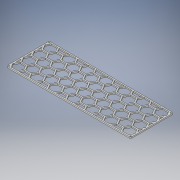
# Autodesk Inventor part: plate
Saved by Autodesk Inventor 2019 (Build 230136000, 136)
## iProperties
Created: 2019-01-24
Part Number: plate
Material: Generic
Document SubType Name: Modeling
Designer: Andrew
Density: 1 g/cm^3
Appearance: Default
Author: Andrew
Autodesk Inventor part; units mm, degrees
ref_plane "YZ Plane" through (0, 0, 0) normal (1, 0, 0) x (0, 1, 0)
ref_plane "XZ Plane" through (0, 0, 0) normal (0, 1, 0) x (-1, 0, 0)
ref_plane "XY Plane" through (0, 0, 0) normal (0, 0, 1) x (1, 0, 0)
sketch "Sketch1" plane through (0, 0, 0) normal (0, 1, 0) x (-1, 0, 0)
  line L0 (290.7004, 97.1993) -> (290.7004, 3)
  arc A0 (287.7004, 0) -> (290.7004, 3) centre (287.7004, 3) ccw
  arc A1 (290.7004, 97.1993) -> (287.7004, 100.1993) centre (287.7004, 97.1993) ccw
  line L1 (3, 0) -> (287.7004, 0)
  line L2 (0, 97.1993) -> (0, 3)
  line L3 (287.7004, 100.1993) -> (3, 100.1993)
  arc A2 (3, 100.1993) -> (0, 97.1993) centre (3, 97.1993) ccw
  circle A3 centre (287.7004, 97.1993) radius 1.5
  circle A4 centre (3, 97.1993) radius 1.5
  circle A5 centre (3, 3) radius 1.5
  circle A6 centre (287.7004, 3) radius 1.5
  line L4 (3, 88.615) -> (3, 86.7338)
  line L5 (7.9562, 3) -> (22.4187, 3)
  line L6 (287.7004, 88.615) -> (287.7004, 86.7338)
  line L7 (282.7442, 97.1993) -> (268.2817, 97.1993)
  arc A7 (0, 3) -> (3, 0) centre (3, 3) ccw
  line L8 (30.516, 86.1744) -> (24.1507, 75.1495)
  line L9 (30.516, 86.1744) -> (43.2465, 86.1744)
  line L10 (43.2465, 86.1744) -> (49.6117, 75.1495)
  line L11 (49.6117, 75.1495) -> (43.2465, 64.1246)
  line L12 (30.516, 64.1246) -> (43.2465, 64.1246)
  line L13 (24.1507, 75.1495) -> (30.516, 64.1246)
  line L14 (52.2098, 73.6495) -> (45.8445, 62.6246)
  line L15 (45.8445, 62.6246) -> (52.2098, 51.5997)
  line L16 (71.3055, 62.6246) -> (64.9402, 51.5997)
  line L17 (64.9402, 73.6495) -> (71.3055, 62.6246)
  line L18 (52.2098, 51.5997) -> (64.9402, 51.5997)
  line L19 (52.2098, 73.6495) -> (64.9402, 73.6495)
  line L20 (73.9036, 86.1744) -> (67.5383, 75.1495)
  line L21 (67.5383, 75.1495) -> (73.9036, 64.1246)
  line L22 (92.9993, 75.1495) -> (86.634, 64.1246)
  line L23 (86.634, 86.1744) -> (92.9993, 75.1495)
  line L24 (73.9036, 64.1246) -> (86.634, 64.1246)
  line L25 (73.9036, 86.1744) -> (86.634, 86.1744)
  line L26 (95.5974, 73.6495) -> (89.2321, 62.6246)
  line L27 (89.2321, 62.6246) -> (95.5974, 51.5997)
  line L28 (114.6931, 62.6246) -> (108.3278, 51.5997)
  line L29 (108.3278, 73.6495) -> (114.6931, 62.6246)
  line L30 (95.5974, 51.5997) -> (108.3278, 51.5997)
  line L31 (95.5974, 73.6495) -> (108.3278, 73.6495)
  line L32 (73.9036, 61.1246) -> (67.5383, 50.0997)
  line L33 (67.5383, 50.0997) -> (73.9036, 39.0747)
  line L34 (92.9993, 50.0997) -> (86.634, 39.0747)
  line L35 (86.634, 61.1246) -> (92.9993, 50.0997)
  line L36 (73.9036, 39.0747) -> (86.634, 39.0747)
  line L37 (73.9036, 61.1246) -> (86.634, 61.1246)
  line L38 (52.2098, 48.5997) -> (45.8445, 37.5747)
  line L39 (45.8445, 37.5747) -> (52.2098, 26.5498)
  line L40 (71.3055, 37.5747) -> (64.9402, 26.5498)
  line L41 (64.9402, 48.5997) -> (71.3055, 37.5747)
  line L42 (52.2098, 26.5498) -> (64.9402, 26.5498)
  line L43 (52.2098, 48.5997) -> (64.9402, 48.5997)
  line L44 (73.9036, 36.0747) -> (67.5383, 25.0498)
  line L45 (67.5383, 25.0498) -> (73.9036, 14.0249)
  line L46 (92.9993, 25.0498) -> (86.634, 14.0249)
  line L47 (86.634, 36.0747) -> (92.9993, 25.0498)
  line L48 (73.9036, 14.0249) -> (86.634, 14.0249)
  line L49 (73.9036, 36.0747) -> (86.634, 36.0747)
  line L50 (95.5974, 48.5997) -> (89.2321, 37.5747)
  line L51 (89.2321, 37.5747) -> (95.5974, 26.5498)
  line L52 (114.6931, 37.5747) -> (108.3278, 26.5498)
  line L53 (108.3278, 48.5997) -> (114.6931, 37.5747)
  line L54 (95.5974, 26.5498) -> (108.3278, 26.5498)
  line L55 (95.5974, 48.5997) -> (108.3278, 48.5997)
  line L56 (117.2911, 61.1246) -> (110.9259, 50.0997)
  line L57 (110.9259, 50.0997) -> (117.2911, 39.0747)
  line L58 (136.3869, 50.0997) -> (130.0216, 39.0747)
  line L59 (130.0216, 61.1246) -> (136.3869, 50.0997)
  line L60 (117.2911, 39.0747) -> (130.0216, 39.0747)
  line L61 (117.2911, 61.1246) -> (130.0216, 61.1246)
  line L62 (138.9849, 73.6495) -> (132.6197, 62.6246)
  line L63 (132.6197, 62.6246) -> (138.9849, 51.5997)
  line L64 (158.0807, 62.6246) -> (151.7154, 51.5997)
  line L65 (151.7154, 73.6495) -> (158.0807, 62.6246)
  line L66 (138.9849, 51.5997) -> (151.7154, 51.5997)
  line L67 (138.9849, 73.6495) -> (151.7154, 73.6495)
  line L68 (160.6787, 61.1246) -> (154.3135, 50.0997)
  line L69 (154.3135, 50.0997) -> (160.6787, 39.0747)
  line L70 (179.7744, 50.0997) -> (173.4092, 39.0747)
  line L71 (173.4092, 61.1246) -> (179.7744, 50.0997)
  line L72 (160.6787, 39.0747) -> (173.4092, 39.0747)
  line L73 (160.6787, 61.1246) -> (173.4092, 61.1246)
  line L74 (138.9849, 48.5997) -> (132.6197, 37.5747)
  line L75 (132.6197, 37.5747) -> (138.9849, 26.5498)
  line L76 (158.0807, 37.5747) -> (151.7154, 26.5498)
  line L77 (151.7154, 48.5997) -> (158.0807, 37.5747)
  line L78 (138.9849, 26.5498) -> (151.7154, 26.5498)
  line L79 (138.9849, 48.5997) -> (151.7154, 48.5997)
  line L80 (117.2911, 36.0747) -> (110.9259, 25.0498)
  line L81 (110.9259, 25.0498) -> (117.2911, 14.0249)
  line L82 (136.3869, 25.0498) -> (130.0216, 14.0249)
  line L83 (130.0216, 36.0747) -> (136.3869, 25.0498)
  line L84 (117.2911, 14.0249) -> (130.0216, 14.0249)
  line L85 (117.2911, 36.0747) -> (130.0216, 36.0747)
  line L86 (160.6787, 36.0747) -> (154.3135, 25.0498)
  line L87 (154.3135, 25.0498) -> (160.6787, 14.0249)
  line L88 (179.7744, 25.0498) -> (173.4092, 14.0249)
  line L89 (173.4092, 36.0747) -> (179.7744, 25.0498)
  line L90 (160.6787, 14.0249) -> (173.4092, 14.0249)
  line L91 (160.6787, 36.0747) -> (173.4092, 36.0747)
  line L92 (182.3725, 48.5997) -> (176.0073, 37.5747)
  line L93 (176.0073, 37.5747) -> (182.3725, 26.5498)
  line L94 (201.4682, 37.5747) -> (195.103, 26.5498)
  line L95 (195.103, 48.5997) -> (201.4682, 37.5747)
  line L96 (182.3725, 26.5498) -> (195.103, 26.5498)
  line L97 (182.3725, 48.5997) -> (195.103, 48.5997)
  line L98 (182.3725, 73.6495) -> (176.0073, 62.6246)
  line L99 (176.0073, 62.6246) -> (182.3725, 51.5997)
  line L100 (201.4682, 62.6246) -> (195.103, 51.5997)
  line L101 (195.103, 73.6495) -> (201.4682, 62.6246)
  line L102 (182.3725, 51.5997) -> (195.103, 51.5997)
  line L103 (182.3725, 73.6495) -> (195.103, 73.6495)
  line L104 (160.6787, 86.1744) -> (154.3135, 75.1495)
  line L105 (154.3135, 75.1495) -> (160.6787, 64.1246)
  line L106 (179.7744, 75.1495) -> (173.4092, 64.1246)
  line L107 (173.4092, 86.1744) -> (179.7744, 75.1495)
  line L108 (160.6787, 64.1246) -> (173.4092, 64.1246)
  line L109 (160.6787, 86.1744) -> (173.4092, 86.1744)
  line L110 (204.0663, 86.1744) -> (197.7011, 75.1495)
  line L111 (197.7011, 75.1495) -> (204.0663, 64.1246)
  line L112 (223.162, 75.1495) -> (216.7968, 64.1246)
  line L113 (216.7968, 86.1744) -> (223.162, 75.1495)
  line L114 (204.0663, 64.1246) -> (216.7968, 64.1246)
  line L115 (204.0663, 86.1744) -> (216.7968, 86.1744)
  line L116 (204.0663, 61.1246) -> (197.7011, 50.0997)
  line L117 (197.7011, 50.0997) -> (204.0663, 39.0747)
  line L118 (223.162, 50.0997) -> (216.7968, 39.0747)
  line L119 (216.7968, 61.1246) -> (223.162, 50.0997)
  line L120 (204.0663, 39.0747) -> (216.7968, 39.0747)
  line L121 (204.0663, 61.1246) -> (216.7968, 61.1246)
  line L122 (225.7601, 73.6495) -> (219.3949, 62.6246)
  line L123 (219.3949, 62.6246) -> (225.7601, 51.5997)
  line L124 (244.8558, 62.6246) -> (238.4906, 51.5997)
  line L125 (238.4906, 73.6495) -> (244.8558, 62.6246)
  line L126 (225.7601, 51.5997) -> (238.4906, 51.5997)
  line L127 (225.7601, 73.6495) -> (238.4906, 73.6495)
  line L128 (225.7601, 48.5997) -> (219.3949, 37.5747)
  line L129 (219.3949, 37.5747) -> (225.7601, 26.5498)
  line L130 (244.8558, 37.5747) -> (238.4906, 26.5498)
  line L131 (238.4906, 48.5997) -> (244.8558, 37.5747)
  line L132 (225.7601, 26.5498) -> (238.4906, 26.5498)
  line L133 (225.7601, 48.5997) -> (238.4906, 48.5997)
  line L134 (204.0663, 36.0747) -> (197.7011, 25.0498)
  line L135 (197.7011, 25.0498) -> (204.0663, 14.0249)
  line L136 (223.162, 25.0498) -> (216.7968, 14.0249)
  line L137 (216.7968, 36.0747) -> (223.162, 25.0498)
  line L138 (204.0663, 14.0249) -> (216.7968, 14.0249)
  line L139 (204.0663, 36.0747) -> (216.7968, 36.0747)
  line L140 (247.4539, 36.0747) -> (241.0887, 25.0498)
  line L141 (241.0887, 25.0498) -> (247.4539, 14.0249)
  line L142 (266.5496, 25.0498) -> (260.1844, 14.0249)
  line L143 (260.1844, 36.0747) -> (266.5496, 25.0498)
  line L144 (247.4539, 14.0249) -> (260.1844, 14.0249)
  line L145 (247.4539, 36.0747) -> (260.1844, 36.0747)
  line L146 (247.4539, 61.1246) -> (241.0887, 50.0997)
  line L147 (241.0887, 50.0997) -> (247.4539, 39.0747)
  line L148 (266.5496, 50.0997) -> (260.1844, 39.0747)
  line L149 (260.1844, 61.1246) -> (266.5496, 50.0997)
  line L150 (247.4539, 39.0747) -> (260.1844, 39.0747)
  line L151 (247.4539, 61.1246) -> (260.1844, 61.1246)
  line L152 (247.4539, 86.1744) -> (241.0887, 75.1495)
  line L153 (241.0887, 75.1495) -> (247.4539, 64.1246)
  line L154 (266.5496, 75.1495) -> (260.1844, 64.1246)
  line L155 (260.1844, 86.1744) -> (266.5496, 75.1495)
  line L156 (247.4539, 64.1246) -> (260.1844, 64.1246)
  line L157 (247.4539, 86.1744) -> (260.1844, 86.1744)
  line L158 (30.516, 61.1246) -> (24.1507, 50.0997)
  line L159 (24.1507, 50.0997) -> (30.516, 39.0747)
  line L160 (49.6117, 50.0997) -> (43.2465, 39.0747)
  line L161 (43.2465, 61.1246) -> (49.6117, 50.0997)
  line L162 (30.516, 39.0747) -> (43.2465, 39.0747)
  line L163 (30.516, 61.1246) -> (43.2465, 61.1246)
  line L164 (30.516, 36.0747) -> (24.1507, 25.0498)
  line L165 (24.1507, 25.0498) -> (30.516, 14.0249)
  line L166 (49.6117, 25.0498) -> (43.2465, 14.0249)
  line L167 (43.2465, 36.0747) -> (49.6117, 25.0498)
  line L168 (30.516, 14.0249) -> (43.2465, 14.0249)
  line L169 (30.516, 36.0747) -> (43.2465, 36.0747)
  line L170 (8.8222, 73.6495) -> (3, 63.5652)
  line L171 (3, 61.684) -> (8.8222, 51.5997)
  line L172 (27.9179, 62.6246) -> (21.5527, 51.5997)
  line L173 (21.5527, 73.6495) -> (27.9179, 62.6246)
  line L174 (8.8222, 51.5997) -> (21.5527, 51.5997)
  line L175 (8.8222, 73.6495) -> (21.5527, 73.6495)
  line L176 (7.9562, 97.1993) -> (3, 88.615)
  line L177 (3, 86.7338) -> (8.8222, 76.6495)
  line L178 (27.9179, 87.6744) -> (21.5527, 76.6495)
  line L179 (22.4187, 97.1993) -> (27.9179, 87.6744)
  line L180 (8.8222, 76.6495) -> (21.5527, 76.6495)
  line L181 (8.8222, 48.5997) -> (3, 38.5153)
  line L182 (3, 36.6342) -> (8.8222, 26.5498)
  line L183 (27.9179, 37.5747) -> (21.5527, 26.5498)
  line L184 (21.5527, 48.5997) -> (27.9179, 37.5747)
  line L185 (8.8222, 26.5498) -> (21.5527, 26.5498)
  line L186 (8.8222, 48.5997) -> (21.5527, 48.5997)
  line L187 (25.8828, 97.1993) -> (30.516, 89.1744)
  line L188 (47.8796, 97.1993) -> (43.2465, 89.1744)
  line L189 (30.516, 89.1744) -> (43.2465, 89.1744)
  line L190 (69.2704, 97.1993) -> (73.9036, 89.1744)
  line L191 (91.2672, 97.1993) -> (86.634, 89.1744)
  line L192 (73.9036, 89.1744) -> (86.634, 89.1744)
  line L193 (112.658, 97.1993) -> (117.2911, 89.1744)
  line L194 (134.6548, 97.1993) -> (130.0216, 89.1744)
  line L195 (117.2911, 89.1744) -> (130.0216, 89.1744)
  line L196 (156.0455, 97.1993) -> (160.6787, 89.1744)
  line L197 (178.0424, 97.1993) -> (173.4092, 89.1744)
  line L198 (160.6787, 89.1744) -> (173.4092, 89.1744)
  line L199 (199.4331, 97.1993) -> (204.0663, 89.1744)
  line L200 (221.43, 97.1993) -> (216.7968, 89.1744)
  line L201 (204.0663, 89.1744) -> (216.7968, 89.1744)
  line L202 (242.8207, 97.1993) -> (247.4539, 89.1744)
  line L203 (264.8176, 97.1993) -> (260.1844, 89.1744)
  line L204 (247.4539, 89.1744) -> (260.1844, 89.1744)
  line L205 (224.8941, 97.1993) -> (219.3949, 87.6744)
  line L206 (219.3949, 87.6744) -> (225.7601, 76.6495)
  line L207 (244.8558, 87.6744) -> (238.4906, 76.6495)
  line L208 (239.3566, 97.1993) -> (244.8558, 87.6744)
  line L209 (225.7601, 76.6495) -> (238.4906, 76.6495)
  line L210 (181.5065, 97.1993) -> (176.0073, 87.6744)
  line L211 (176.0073, 87.6744) -> (182.3725, 76.6495)
  line L212 (201.4682, 87.6744) -> (195.103, 76.6495)
  line L213 (195.969, 97.1993) -> (201.4682, 87.6744)
  line L214 (182.3725, 76.6495) -> (195.103, 76.6495)
  line L215 (138.1189, 97.1993) -> (132.6197, 87.6744)
  line L216 (132.6197, 87.6744) -> (138.9849, 76.6495)
  line L217 (158.0807, 87.6744) -> (151.7154, 76.6495)
  line L218 (152.5814, 97.1993) -> (158.0807, 87.6744)
  line L219 (138.9849, 76.6495) -> (151.7154, 76.6495)
  line L220 (94.7313, 97.1993) -> (89.2321, 87.6744)
  line L221 (89.2321, 87.6744) -> (95.5974, 76.6495)
  line L222 (114.6931, 87.6744) -> (108.3278, 76.6495)
  line L223 (109.1939, 97.1993) -> (114.6931, 87.6744)
  line L224 (95.5974, 76.6495) -> (108.3278, 76.6495)
  line L225 (117.2911, 86.1744) -> (110.9259, 75.1495)
  line L226 (110.9259, 75.1495) -> (117.2911, 64.1246)
  line L227 (136.3869, 75.1495) -> (130.0216, 64.1246)
  line L228 (130.0216, 86.1744) -> (136.3869, 75.1495)
  line L229 (117.2911, 64.1246) -> (130.0216, 64.1246)
  line L230 (117.2911, 86.1744) -> (130.0216, 86.1744)
  line L231 (51.3437, 97.1993) -> (45.8445, 87.6744)
  line L232 (45.8445, 87.6744) -> (52.2098, 76.6495)
  line L233 (71.3055, 87.6744) -> (64.9402, 76.6495)
  line L234 (65.8063, 97.1993) -> (71.3055, 87.6744)
  line L235 (52.2098, 76.6495) -> (64.9402, 76.6495)
  line L236 (268.2817, 97.1993) -> (262.7824, 87.6744)
  line L237 (262.7824, 87.6744) -> (269.1477, 76.6495)
  line L238 (287.7004, 86.7338) -> (281.8782, 76.6495)
  line L239 (282.7442, 97.1993) -> (287.7004, 88.615)
  line L240 (269.1477, 76.6495) -> (281.8782, 76.6495)
  line L241 (269.1477, 73.6495) -> (262.7824, 62.6246)
  line L242 (262.7824, 62.6246) -> (269.1477, 51.5997)
  line L243 (287.7004, 61.684) -> (281.8782, 51.5997)
  line L244 (281.8782, 73.6495) -> (287.7004, 63.5652)
  line L245 (269.1477, 51.5997) -> (281.8782, 51.5997)
  line L246 (269.1477, 73.6495) -> (281.8782, 73.6495)
  line L247 (269.1477, 48.5997) -> (262.7824, 37.5747)
  line L248 (262.7824, 37.5747) -> (269.1477, 26.5498)
  line L249 (287.7004, 36.6342) -> (281.8782, 26.5498)
  line L250 (281.8782, 48.5997) -> (287.7004, 38.5153)
  line L251 (269.1477, 26.5498) -> (281.8782, 26.5498)
  line L252 (269.1477, 48.5997) -> (281.8782, 48.5997)
  line L253 (8.8222, 23.5498) -> (3, 13.4655)
  line L254 (3, 11.5843) -> (7.9562, 3)
  line L255 (27.9179, 12.5249) -> (22.4187, 3)
  line L256 (21.5527, 23.5498) -> (27.9179, 12.5249)
  line L257 (8.8222, 23.5498) -> (21.5527, 23.5498)
  line L258 (30.516, 11.0249) -> (25.8828, 3)
  line L259 (43.2465, 11.0249) -> (47.8796, 3)
  line L260 (30.516, 11.0249) -> (43.2465, 11.0249)
  line L261 (52.2098, 23.5498) -> (45.8445, 12.5249)
  line L262 (45.8445, 12.5249) -> (51.3437, 3)
  line L263 (71.3055, 12.5249) -> (65.8063, 3)
  line L264 (64.9402, 23.5498) -> (71.3055, 12.5249)
  line L265 (52.2098, 23.5498) -> (64.9402, 23.5498)
  line L266 (73.9036, 11.0249) -> (69.2704, 3)
  line L267 (86.634, 11.0249) -> (91.2672, 3)
  line L268 (73.9036, 11.0249) -> (86.634, 11.0249)
  line L269 (95.5974, 23.5498) -> (89.2321, 12.5249)
  line L270 (89.2321, 12.5249) -> (94.7313, 3)
  line L271 (114.6931, 12.5249) -> (109.1939, 3)
  line L272 (108.3278, 23.5498) -> (114.6931, 12.5249)
  line L273 (95.5974, 23.5498) -> (108.3278, 23.5498)
  line L274 (138.9849, 23.5498) -> (132.6197, 12.5249)
  line L275 (132.6197, 12.5249) -> (138.1189, 3)
  line L276 (158.0807, 12.5249) -> (152.5814, 3)
  line L277 (151.7154, 23.5498) -> (158.0807, 12.5249)
  line L278 (138.9849, 23.5498) -> (151.7154, 23.5498)
  line L279 (117.2911, 11.0249) -> (112.658, 3)
  line L280 (130.0216, 11.0249) -> (134.6548, 3)
  line L281 (117.2911, 11.0249) -> (130.0216, 11.0249)
  line L282 (160.6787, 11.0249) -> (156.0455, 3)
  line L283 (173.4092, 11.0249) -> (178.0424, 3)
  line L284 (160.6787, 11.0249) -> (173.4092, 11.0249)
  line L285 (182.3725, 23.5498) -> (176.0073, 12.5249)
  line L286 (176.0073, 12.5249) -> (181.5065, 3)
  line L287 (201.4682, 12.5249) -> (195.969, 3)
  line L288 (195.103, 23.5498) -> (201.4682, 12.5249)
  line L289 (182.3725, 23.5498) -> (195.103, 23.5498)
  line L290 (204.0663, 11.0249) -> (199.4331, 3)
  line L291 (216.7968, 11.0249) -> (221.43, 3)
  line L292 (204.0663, 11.0249) -> (216.7968, 11.0249)
  line L293 (225.7601, 23.5498) -> (219.3949, 12.5249)
  line L294 (219.3949, 12.5249) -> (224.8941, 3)
  line L295 (244.8558, 12.5249) -> (239.3566, 3)
  line L296 (238.4906, 23.5498) -> (244.8558, 12.5249)
  line L297 (225.7601, 23.5498) -> (238.4906, 23.5498)
  line L298 (247.4539, 11.0249) -> (242.8207, 3)
  line L299 (260.1844, 11.0249) -> (264.8176, 3)
  line L300 (247.4539, 11.0249) -> (260.1844, 11.0249)
  line L301 (269.1477, 23.5498) -> (262.7824, 12.5249)
  line L302 (262.7824, 12.5249) -> (268.2817, 3)
  line L303 (287.7004, 11.5843) -> (282.7442, 3)
  line L304 (281.8782, 23.5498) -> (287.7004, 13.4655)
  line L305 (269.1477, 23.5498) -> (281.8782, 23.5498)
  line L306 (6.2241, 75.1495) -> (3, 69.5652)
  line L307 (3, 80.7338) -> (6.2241, 75.1495)
  line L308 (6.2241, 50.0997) -> (3, 44.5153)
  line L309 (3, 55.684) -> (6.2241, 50.0997)
  line L310 (3, 30.6342) -> (6.2241, 25.0498)
  line L311 (6.2241, 25.0498) -> (3, 19.4655)
  line L312 (287.7004, 80.7338) -> (284.4762, 75.1495)
  line L313 (284.4762, 75.1495) -> (287.7004, 69.5652)
  line L314 (287.7004, 55.684) -> (284.4762, 50.0997)
  line L315 (284.4762, 50.0997) -> (287.7004, 44.5153)
  line L316 (284.4762, 25.0498) -> (287.7004, 19.4655)
  line L317 (287.7004, 30.6342) -> (284.4762, 25.0498)
  line L318 (22.4187, 97.1993) -> (7.9562, 97.1993)
  line L319 (47.8796, 97.1993) -> (25.8828, 97.1993)
  line L320 (65.8063, 97.1993) -> (51.3437, 97.1993)
  line L321 (91.2672, 97.1993) -> (69.2704, 97.1993)
  line L322 (109.1939, 97.1993) -> (94.7313, 97.1993)
  line L323 (134.6548, 97.1993) -> (112.658, 97.1993)
  line L324 (152.5814, 97.1993) -> (138.1189, 97.1993)
  line L325 (178.0424, 97.1993) -> (156.0455, 97.1993)
  line L326 (195.969, 97.1993) -> (181.5065, 97.1993)
  line L327 (239.3566, 97.1993) -> (224.8941, 97.1993)
  line L328 (221.43, 97.1993) -> (199.4331, 97.1993)
  line L329 (264.8176, 97.1993) -> (242.8207, 97.1993)
  line L330 (287.7004, 80.7338) -> (287.7004, 69.5652)
  line L331 (287.7004, 63.5652) -> (287.7004, 61.684)
  line L332 (287.7004, 38.5153) -> (287.7004, 36.6342)
  line L333 (287.7004, 55.684) -> (287.7004, 44.5153)
  line L334 (287.7004, 30.6342) -> (287.7004, 19.4655)
  line L335 (287.7004, 13.4655) -> (287.7004, 11.5843)
  line L336 (268.2817, 3) -> (282.7442, 3)
  line L337 (242.8207, 3) -> (264.8176, 3)
  line L338 (224.8941, 3) -> (239.3566, 3)
  line L339 (199.4331, 3) -> (221.43, 3)
  line L340 (181.5065, 3) -> (195.969, 3)
  line L341 (156.0455, 3) -> (178.0424, 3)
  line L342 (138.1189, 3) -> (152.5814, 3)
  line L343 (112.658, 3) -> (134.6548, 3)
  line L344 (94.7313, 3) -> (109.1939, 3)
  line L345 (69.2704, 3) -> (91.2672, 3)
  line L346 (51.3437, 3) -> (65.8063, 3)
  line L347 (25.8828, 3) -> (47.8796, 3)
  line L348 (3, 13.4655) -> (3, 11.5843)
  line L349 (3, 30.6342) -> (3, 19.4655)
  line L350 (3, 38.5153) -> (3, 36.6342)
  line L351 (3, 55.684) -> (3, 44.5153)
  line L352 (3, 63.5652) -> (3, 61.684)
  line L353 (3, 80.7338) -> (3, 69.5652)
  line L354 (247.4539, 61.1246) -> (241.0887, 50.0997)
  line L355 (241.0887, 50.0997) -> (247.4539, 39.0747)
  line L356 (266.5496, 50.0997) -> (260.1844, 39.0747)
  line L357 (260.1844, 61.1246) -> (266.5496, 50.0997)
  line L358 (247.4539, 39.0747) -> (260.1844, 39.0747)
  line L359 (247.4539, 61.1246) -> (260.1844, 61.1246)
  line L360 (247.4539, 86.1744) -> (241.0887, 75.1495)
  line L361 (241.0887, 75.1495) -> (247.4539, 64.1246)
  line L362 (266.5496, 75.1495) -> (260.1844, 64.1246)
  line L363 (260.1844, 86.1744) -> (266.5496, 75.1495)
  line L364 (247.4539, 64.1246) -> (260.1844, 64.1246)
  line L365 (247.4539, 86.1744) -> (260.1844, 86.1744)
  line L366 (225.7601, 73.6495) -> (219.3949, 62.6246)
  line L367 (219.3949, 62.6246) -> (225.7601, 51.5997)
  line L368 (244.8558, 62.6246) -> (238.4906, 51.5997)
  line L369 (238.4906, 73.6495) -> (244.8558, 62.6246)
  line L370 (225.7601, 51.5997) -> (238.4906, 51.5997)
  line L371 (225.7601, 73.6495) -> (238.4906, 73.6495)
  line L372 (225.7601, 48.5997) -> (219.3949, 37.5747)
  line L373 (219.3949, 37.5747) -> (225.7601, 26.5498)
  line L374 (244.8558, 37.5747) -> (238.4906, 26.5498)
  line L375 (238.4906, 48.5997) -> (244.8558, 37.5747)
  line L376 (225.7601, 26.5498) -> (238.4906, 26.5498)
  line L377 (225.7601, 48.5997) -> (238.4906, 48.5997)
  line L378 (204.0663, 36.0747) -> (197.7011, 25.0498)
  line L379 (197.7011, 25.0498) -> (204.0663, 14.0249)
  line L380 (223.162, 25.0498) -> (216.7968, 14.0249)
  line L381 (216.7968, 36.0747) -> (223.162, 25.0498)
  line L382 (204.0663, 14.0249) -> (216.7968, 14.0249)
  line L383 (204.0663, 36.0747) -> (216.7968, 36.0747)
  line L384 (204.0663, 61.1246) -> (197.7011, 50.0997)
  line L385 (197.7011, 50.0997) -> (204.0663, 39.0747)
  line L386 (223.162, 50.0997) -> (216.7968, 39.0747)
  line L387 (216.7968, 61.1246) -> (223.162, 50.0997)
  line L388 (204.0663, 39.0747) -> (216.7968, 39.0747)
  line L389 (204.0663, 61.1246) -> (216.7968, 61.1246)
  line L390 (204.0663, 86.1744) -> (197.7011, 75.1495)
  line L391 (197.7011, 75.1495) -> (204.0663, 64.1246)
  line L392 (223.162, 75.1495) -> (216.7968, 64.1246)
  line L393 (216.7968, 86.1744) -> (223.162, 75.1495)
  line L394 (204.0663, 64.1246) -> (216.7968, 64.1246)
  line L395 (204.0663, 86.1744) -> (216.7968, 86.1744)
  line L396 (182.3725, 73.6495) -> (176.0073, 62.6246)
  line L397 (176.0073, 62.6246) -> (182.3725, 51.5997)
  line L398 (201.4682, 62.6246) -> (195.103, 51.5997)
  line L399 (195.103, 73.6495) -> (201.4682, 62.6246)
  line L400 (182.3725, 51.5997) -> (195.103, 51.5997)
  line L401 (182.3725, 73.6495) -> (195.103, 73.6495)
  line L402 (182.3725, 48.5997) -> (176.0073, 37.5747)
  line L403 (176.0073, 37.5747) -> (182.3725, 26.5498)
  line L404 (201.4682, 37.5747) -> (195.103, 26.5498)
  line L405 (195.103, 48.5997) -> (201.4682, 37.5747)
  line L406 (182.3725, 26.5498) -> (195.103, 26.5498)
  line L407 (182.3725, 48.5997) -> (195.103, 48.5997)
  line L408 (160.6787, 36.0747) -> (154.3135, 25.0498)
  line L409 (154.3135, 25.0498) -> (160.6787, 14.0249)
  line L410 (179.7744, 25.0498) -> (173.4092, 14.0249)
  line L411 (173.4092, 36.0747) -> (179.7744, 25.0498)
  line L412 (160.6787, 14.0249) -> (173.4092, 14.0249)
  line L413 (160.6787, 36.0747) -> (173.4092, 36.0747)
  line L414 (160.6787, 61.1246) -> (154.3135, 50.0997)
  line L415 (154.3135, 50.0997) -> (160.6787, 39.0747)
  line L416 (179.7744, 50.0997) -> (173.4092, 39.0747)
  line L417 (173.4092, 61.1246) -> (179.7744, 50.0997)
  line L418 (160.6787, 39.0747) -> (173.4092, 39.0747)
  line L419 (160.6787, 61.1246) -> (173.4092, 61.1246)
  line L420 (160.6787, 86.1744) -> (154.3135, 75.1495)
  line L421 (154.3135, 75.1495) -> (160.6787, 64.1246)
  line L422 (179.7744, 75.1495) -> (173.4092, 64.1246)
  line L423 (173.4092, 86.1744) -> (179.7744, 75.1495)
  line L424 (160.6787, 64.1246) -> (173.4092, 64.1246)
  line L425 (160.6787, 86.1744) -> (173.4092, 86.1744)
  line L426 (138.9849, 73.6495) -> (132.6197, 62.6246)
  line L427 (132.6197, 62.6246) -> (138.9849, 51.5997)
  line L428 (158.0807, 62.6246) -> (151.7154, 51.5997)
  line L429 (151.7154, 73.6495) -> (158.0807, 62.6246)
  line L430 (138.9849, 51.5997) -> (151.7154, 51.5997)
  line L431 (138.9849, 73.6495) -> (151.7154, 73.6495)
  line L432 (138.9849, 48.5997) -> (132.6197, 37.5747)
  line L433 (132.6197, 37.5747) -> (138.9849, 26.5498)
  line L434 (158.0807, 37.5747) -> (151.7154, 26.5498)
  line L435 (151.7154, 48.5997) -> (158.0807, 37.5747)
  line L436 (138.9849, 26.5498) -> (151.7154, 26.5498)
  line L437 (138.9849, 48.5997) -> (151.7154, 48.5997)
  line L438 (117.2911, 36.0747) -> (110.9259, 25.0498)
  line L439 (110.9259, 25.0498) -> (117.2911, 14.0249)
  line L440 (136.3869, 25.0498) -> (130.0216, 14.0249)
  line L441 (130.0216, 36.0747) -> (136.3869, 25.0498)
  line L442 (117.2911, 14.0249) -> (130.0216, 14.0249)
  line L443 (117.2911, 36.0747) -> (130.0216, 36.0747)
  line L444 (117.2911, 61.1246) -> (110.9259, 50.0997)
  line L445 (110.9259, 50.0997) -> (117.2911, 39.0747)
  line L446 (136.3869, 50.0997) -> (130.0216, 39.0747)
  line L447 (130.0216, 61.1246) -> (136.3869, 50.0997)
  line L448 (117.2911, 39.0747) -> (130.0216, 39.0747)
  line L449 (117.2911, 61.1246) -> (130.0216, 61.1246)
  line L450 (117.2911, 86.1744) -> (110.9259, 75.1495)
  line L451 (110.9259, 75.1495) -> (117.2911, 64.1246)
  line L452 (136.3869, 75.1495) -> (130.0216, 64.1246)
  line L453 (130.0216, 86.1744) -> (136.3869, 75.1495)
  line L454 (117.2911, 64.1246) -> (130.0216, 64.1246)
  line L455 (117.2911, 86.1744) -> (130.0216, 86.1744)
  line L456 (95.5974, 73.6495) -> (89.2321, 62.6246)
  line L457 (89.2321, 62.6246) -> (95.5974, 51.5997)
  line L458 (114.6931, 62.6246) -> (108.3278, 51.5997)
  line L459 (108.3278, 73.6495) -> (114.6931, 62.6246)
  line L460 (95.5974, 51.5997) -> (108.3278, 51.5997)
  line L461 (95.5974, 73.6495) -> (108.3278, 73.6495)
  line L462 (95.5974, 48.5997) -> (89.2321, 37.5747)
  line L463 (89.2321, 37.5747) -> (95.5974, 26.5498)
  line L464 (114.6931, 37.5747) -> (108.3278, 26.5498)
  line L465 (108.3278, 48.5997) -> (114.6931, 37.5747)
  line L466 (95.5974, 26.5498) -> (108.3278, 26.5498)
  line L467 (95.5974, 48.5997) -> (108.3278, 48.5997)
  line L468 (73.9036, 36.0747) -> (67.5383, 25.0498)
  line L469 (67.5383, 25.0498) -> (73.9036, 14.0249)
  line L470 (92.9993, 25.0498) -> (86.634, 14.0249)
  line L471 (86.634, 36.0747) -> (92.9993, 25.0498)
  line L472 (73.9036, 14.0249) -> (86.634, 14.0249)
  line L473 (73.9036, 36.0747) -> (86.634, 36.0747)
  line L474 (73.9036, 61.1246) -> (67.5383, 50.0997)
  line L475 (67.5383, 50.0997) -> (73.9036, 39.0747)
  line L476 (92.9993, 50.0997) -> (86.634, 39.0747)
  line L477 (86.634, 61.1246) -> (92.9993, 50.0997)
  line L478 (73.9036, 39.0747) -> (86.634, 39.0747)
  line L479 (73.9036, 61.1246) -> (86.634, 61.1246)
  line L480 (73.9036, 86.1744) -> (67.5383, 75.1495)
  line L481 (67.5383, 75.1495) -> (73.9036, 64.1246)
  line L482 (92.9993, 75.1495) -> (86.634, 64.1246)
  line L483 (86.634, 86.1744) -> (92.9993, 75.1495)
  line L484 (73.9036, 64.1246) -> (86.634, 64.1246)
  line L485 (73.9036, 86.1744) -> (86.634, 86.1744)
  line L486 (52.2098, 73.6495) -> (45.8445, 62.6246)
  line L487 (45.8445, 62.6246) -> (52.2098, 51.5997)
  line L488 (71.3055, 62.6246) -> (64.9402, 51.5997)
  line L489 (64.9402, 73.6495) -> (71.3055, 62.6246)
  line L490 (52.2098, 51.5997) -> (64.9402, 51.5997)
  line L491 (52.2098, 73.6495) -> (64.9402, 73.6495)
  line L492 (52.2098, 48.5997) -> (45.8445, 37.5747)
  line L493 (45.8445, 37.5747) -> (52.2098, 26.5498)
  line L494 (71.3055, 37.5747) -> (64.9402, 26.5498)
  line L495 (64.9402, 48.5997) -> (71.3055, 37.5747)
  line L496 (52.2098, 26.5498) -> (64.9402, 26.5498)
  line L497 (52.2098, 48.5997) -> (64.9402, 48.5997)
  line L498 (30.516, 36.0747) -> (24.1507, 25.0498)
  line L499 (24.1507, 25.0498) -> (30.516, 14.0249)
  line L500 (49.6117, 25.0498) -> (43.2465, 14.0249)
  line L501 (43.2465, 36.0747) -> (49.6117, 25.0498)
  line L502 (30.516, 14.0249) -> (43.2465, 14.0249)
  line L503 (30.516, 36.0747) -> (43.2465, 36.0747)
  line L504 (30.516, 61.1246) -> (24.1507, 50.0997)
  line L505 (24.1507, 50.0997) -> (30.516, 39.0747)
  line L506 (49.6117, 50.0997) -> (43.2465, 39.0747)
  line L507 (43.2465, 61.1246) -> (49.6117, 50.0997)
  line L508 (30.516, 39.0747) -> (43.2465, 39.0747)
  line L509 (30.516, 61.1246) -> (43.2465, 61.1246)
  line L510 (30.516, 86.1744) -> (24.1507, 75.1495)
  line L511 (24.1507, 75.1495) -> (30.516, 64.1246)
  line L512 (49.6117, 75.1495) -> (43.2465, 64.1246)
  line L513 (43.2465, 86.1744) -> (49.6117, 75.1495)
  line L514 (30.516, 64.1246) -> (43.2465, 64.1246)
  line L515 (30.516, 86.1744) -> (43.2465, 86.1744)
  line L516 (269.1477, 73.6495) -> (262.7824, 62.6246)
  line L517 (262.7824, 62.6246) -> (269.1477, 51.5997)
  line L518 (287.7004, 61.684) -> (281.8782, 51.5997)
  line L519 (281.8782, 73.6495) -> (287.7004, 63.5652)
  line L520 (269.1477, 51.5997) -> (281.8782, 51.5997)
  line L521 (269.1477, 73.6495) -> (281.8782, 73.6495)
  line L522 (287.7004, 63.5652) -> (287.7004, 61.684)
  line L523 (181.5065, 97.1993) -> (176.0073, 87.6744)
  line L524 (176.0073, 87.6744) -> (182.3725, 76.6495)
  line L525 (201.4682, 87.6744) -> (195.103, 76.6495)
  line L526 (195.969, 97.1993) -> (201.4682, 87.6744)
  line L527 (182.3725, 76.6495) -> (195.103, 76.6495)
  line L528 (195.969, 97.1993) -> (181.5065, 97.1993)
  line L529 (138.1189, 97.1993) -> (132.6197, 87.6744)
  line L530 (132.6197, 87.6744) -> (138.9849, 76.6495)
  line L531 (158.0807, 87.6744) -> (151.7154, 76.6495)
  line L532 (152.5814, 97.1993) -> (158.0807, 87.6744)
  line L533 (138.9849, 76.6495) -> (151.7154, 76.6495)
  line L534 (152.5814, 97.1993) -> (138.1189, 97.1993)
  line L535 (94.7313, 97.1993) -> (89.2321, 87.6744)
  line L536 (89.2321, 87.6744) -> (95.5974, 76.6495)
  line L537 (114.6931, 87.6744) -> (108.3278, 76.6495)
  line L538 (109.1939, 97.1993) -> (114.6931, 87.6744)
  line L539 (95.5974, 76.6495) -> (108.3278, 76.6495)
  line L540 (109.1939, 97.1993) -> (94.7313, 97.1993)
  line L541 (51.3437, 97.1993) -> (45.8445, 87.6744)
  line L542 (45.8445, 87.6744) -> (52.2098, 76.6495)
  line L543 (71.3055, 87.6744) -> (64.9402, 76.6495)
  line L544 (65.8063, 97.1993) -> (71.3055, 87.6744)
  line L545 (52.2098, 76.6495) -> (64.9402, 76.6495)
  line L546 (65.8063, 97.1993) -> (51.3437, 97.1993)
  line L547 (199.4331, 97.1993) -> (204.0663, 89.1744)
  line L548 (221.43, 97.1993) -> (216.7968, 89.1744)
  line L549 (204.0663, 89.1744) -> (216.7968, 89.1744)
  line L550 (221.43, 97.1993) -> (199.4331, 97.1993)
  line L551 (156.0455, 97.1993) -> (160.6787, 89.1744)
  line L552 (178.0424, 97.1993) -> (173.4092, 89.1744)
  line L553 (160.6787, 89.1744) -> (173.4092, 89.1744)
  line L554 (178.0424, 97.1993) -> (156.0455, 97.1993)
  line L555 (112.658, 97.1993) -> (117.2911, 89.1744)
  line L556 (134.6548, 97.1993) -> (130.0216, 89.1744)
  line L557 (117.2911, 89.1744) -> (130.0216, 89.1744)
  line L558 (134.6548, 97.1993) -> (112.658, 97.1993)
  line L559 (69.2704, 97.1993) -> (73.9036, 89.1744)
  line L560 (91.2672, 97.1993) -> (86.634, 89.1744)
  line L561 (73.9036, 89.1744) -> (86.634, 89.1744)
  line L562 (91.2672, 97.1993) -> (69.2704, 97.1993)
  line L563 (25.8828, 97.1993) -> (30.516, 89.1744)
  line L564 (47.8796, 97.1993) -> (43.2465, 89.1744)
  line L565 (30.516, 89.1744) -> (43.2465, 89.1744)
  line L566 (47.8796, 97.1993) -> (25.8828, 97.1993)
  line L567 (204.0663, 11.0249) -> (199.4331, 3)
  line L568 (216.7968, 11.0249) -> (221.43, 3)
  line L569 (204.0663, 11.0249) -> (216.7968, 11.0249)
  line L570 (199.4331, 3) -> (221.43, 3)
  line L571 (160.6787, 11.0249) -> (156.0455, 3)
  line L572 (173.4092, 11.0249) -> (178.0424, 3)
  line L573 (160.6787, 11.0249) -> (173.4092, 11.0249)
  line L574 (156.0455, 3) -> (178.0424, 3)
  line L575 (117.2911, 11.0249) -> (112.658, 3)
  line L576 (130.0216, 11.0249) -> (134.6548, 3)
  line L577 (117.2911, 11.0249) -> (130.0216, 11.0249)
  line L578 (112.658, 3) -> (134.6548, 3)
  line L579 (73.9036, 11.0249) -> (69.2704, 3)
  line L580 (86.634, 11.0249) -> (91.2672, 3)
  line L581 (73.9036, 11.0249) -> (86.634, 11.0249)
  line L582 (69.2704, 3) -> (91.2672, 3)
  line L583 (30.516, 11.0249) -> (25.8828, 3)
  line L584 (43.2465, 11.0249) -> (47.8796, 3)
  line L585 (30.516, 11.0249) -> (43.2465, 11.0249)
  line L586 (25.8828, 3) -> (47.8796, 3)
  line L587 (182.3725, 23.5498) -> (176.0073, 12.5249)
  line L588 (176.0073, 12.5249) -> (181.5065, 3)
  line L589 (201.4682, 12.5249) -> (195.969, 3)
  line L590 (195.103, 23.5498) -> (201.4682, 12.5249)
  line L591 (182.3725, 23.5498) -> (195.103, 23.5498)
  line L592 (181.5065, 3) -> (195.969, 3)
  line L593 (138.9849, 23.5498) -> (132.6197, 12.5249)
  line L594 (132.6197, 12.5249) -> (138.1189, 3)
  line L595 (158.0807, 12.5249) -> (152.5814, 3)
  line L596 (151.7154, 23.5498) -> (158.0807, 12.5249)
  line L597 (138.9849, 23.5498) -> (151.7154, 23.5498)
  line L598 (138.1189, 3) -> (152.5814, 3)
  line L599 (95.5974, 23.5498) -> (89.2321, 12.5249)
  line L600 (89.2321, 12.5249) -> (94.7313, 3)
  line L601 (114.6931, 12.5249) -> (109.1939, 3)
  line L602 (108.3278, 23.5498) -> (114.6931, 12.5249)
  line L603 (95.5974, 23.5498) -> (108.3278, 23.5498)
  line L604 (94.7313, 3) -> (109.1939, 3)
  line L605 (52.2098, 23.5498) -> (45.8445, 12.5249)
  line L606 (45.8445, 12.5249) -> (51.3437, 3)
  line L607 (71.3055, 12.5249) -> (65.8063, 3)
  line L608 (64.9402, 23.5498) -> (71.3055, 12.5249)
  line L609 (52.2098, 23.5498) -> (64.9402, 23.5498)
  line L610 (51.3437, 3) -> (65.8063, 3)
  point P0 (0, 0)
  constraints: 1222 end point, 8 centre point, 8 point on circle, 1 horizontal
extrude "Extrusion1" add sketch "Sketch1" along normal blind 3
body "Solid1"
